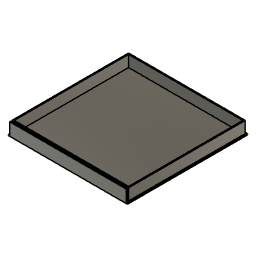
podstawa v2 (Autodesk Fusion 360 design; units mm, degrees)
Autodesk Fusion 360 part; units mm, degrees
sketch "Szkic5" plane through (0, 0, 0) normal (0, 0, 1) x (1, 0, 0)
  line L0 (-100, 100) -> (100, 100)
  line L1 (100, 100) -> (100, -100)
  line L2 (100, -100) -> (-100, -100)
  line L3 (-100, -100) -> (-100, 100)
  line L4 (-102, 102) -> (102, 102)
  line L5 (102, 102) -> (102, -102)
  line L6 (102, -102) -> (-102, -102)
  line L7 (-102, -102) -> (-102, 102)
  line L8 (-104, 104) -> (104, 104)
  line L9 (104, 104) -> (104, -104)
  line L10 (104, -104) -> (-104, -104)
  line L11 (-104, -104) -> (-104, 104)
  line L12 (-106, 106) -> (106, 106)
  line L13 (106, 106) -> (106, -106)
  line L14 (106, -106) -> (-106, -106)
  line L15 (-106, -106) -> (-106, 106)
  line L16 (-104, -104) -> (-104, -106)
  line L17 (104, -104) -> (104, -106)
  line L18 (102, -102) -> (102, -104)
  line L19 (-102, -102) -> (-102, -104)
  line L20 (-102, -104) -> (-102, -106)
  line L21 (104, -104) -> (104, -106)
  line L22 (102, -104) -> (102, -106)
  dimension "d31" = 2
  dimension "d32" = 2
  dimension "d33" = 2
  dimension "d34" = 2
  dimension "d35" = 2
  dimension "d36" = 2
  dimension "d37" = 2
  dimension "d38" = 2
  dimension "d39" = 2
  dimension "d40" = 2
  dimension "d41" = 2
  dimension "d42" = 2
  constraint horizontal L0
  constraint vertical L1
  constraint horizontal L2
  constraint vertical L3
  constraint horizontal L4
  constraint vertical L5
  constraint horizontal L6
  constraint vertical L7
  constraint horizontal L8
  constraint vertical L9
  constraint horizontal L10
  constraint vertical L11
  constraint horizontal L12
  constraint vertical L13
  constraint horizontal L14
  constraint vertical L15
  constraint coincident L14 L16.end
  constraint perpendicular L14 L16
  constraint coincident L14 L17.end
  constraint perpendicular L14 L17
  constraint coincident L10 L18.end
  constraint perpendicular L10 L18
  constraint coincident L10 L19.end
  constraint perpendicular L10 L19
  constraint coincident L14 L20.end
  constraint perpendicular L14 L20
  constraint coincident L14 L22.end
  constraint perpendicular L14 L22
  measures "d31" distance of L2 L6
  measures "d32" distance of L3 L7
  measures "d33" distance of L0 L4
  measures "d34" distance of L1 L5
  measures "d35" distance of L4 L8
  measures "d36" distance of L5 L9
  measures "d37" distance of L6 L10
  measures "d38" distance of L7 L11
  measures "d39" distance of L8 L12
  measures "d40" distance of L9 L13
  measures "d41" distance of L10 L14
  measures "d42" distance of L11 L15
extrude "Wyciągnięcie proste15" add sketch "Szkic5" against normal blind 2 contours L0 L1 L2 L3 | L4 L5 L7 L8 L9 L10 L11 L18 L19 | L4 L5 L6 L7 | L6 L10 L18 L19 | L10 L14 L16 L20 | L10 L14 L20 L22 | L10 L14 L17 L21 L22 | L8 L9 L11 L12 L13 L14 L15 L16 L17 L21
extrude "Wyciągnięcie proste16" add sketch "Szkic5" along normal blind 15 contours L4 L5 L6 L7
extrude "Wyciągnięcie proste17" add sketch "Szkic5" along normal blind 15 contours L10 L14 L16 L20 | L10 L14 L20 L22 | L10 L14 L17 L21 L22
extrude "Wyciągnięcie proste18" cut sketch "Szkic5" against normal blind 2 contours L8 L9 L11 L12 L13 L14 L15 L16 L17 L21
extrude "Extrude19" cut sketch "Szkic5" along normal blind 15 contours L10 L14 L16 L20 | L10 L14 L17 L21 L22
extrude "Extrude20" add 2 faces at (-33.3333, -101.3333, 15) (-34, -105.3333, 15) along direction (0, 0, 1) blind 5
